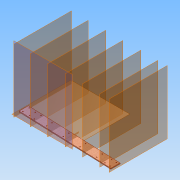
# Autodesk Inventor part: Pancake_Timing Backboard 2
Saved by Autodesk Inventor 2018.1 (Build 221171000, 171)
## iProperties
Created: 2019-02-22
Part Number: Pancake_Timing Backboard 2
Material: Wood (Oak)
Document SubType Name: Modeling
Designer: James
Density: 0.76 g/cm^3
Appearance: White Oak - Natural Medium Gloss
Author: James
Autodesk Inventor part; units mm, degrees
ref_plane "YZ Plane" through (0, 0, 0) normal (1, 0, 0) x (0, 1, 0)
ref_plane "XZ Plane" through (0, 0, 0) normal (0, 1, 0) x (-1, 0, 0)
ref_plane "XY Plane" through (0, 0, 0) normal (0, 0, 1) x (1, 0, 0)
derived "Pancake_Skeleton.ipt"
ref_plane "Ground" through (0, 0, 0) normal (0, 1, 0) x (-1, 0, 0)
ref_plane "Back" through (0, 0, 0) normal (0, 0, 1) x (1, 0, 0)
ref_plane "LHS" through (0, 0, 0) normal (1, 0, 0) x (0, 1, 0)
ref_plane "Lane 1" through (90, 0, 0) normal (1, 0, 0) x (0, 1, 0)
ref_plane "Lane 2" through (185, 0, 0) normal (1, 0, 0) x (0, 1, 0)
ref_plane "Lane 3" through (280, 0, 0) normal (1, 0, 0) x (0, 1, 0)
ref_plane "Lane 4" through (375, 0, 0) normal (1, 0, 0) x (0, 1, 0)
ref_plane "Lane 5" through (470, 0, 0) normal (1, 0, 0) x (0, 1, 0)
ref_plane "RHS" through (520, 0, 0) normal (1, 0, 0) x (0, 1, 0)
sketch "Sketch1" plane through (0, 0, 0) normal (0, 0, 1) x (1, 0, 0)
  line L0 (0, 84) -> (0, -14) projected
  line L1 (520, 84) -> (520, -14) projected
  line L2 (0, 20) -> (520, 0)
  line L3 (520, 0) -> (520, 50)
  line L4 (520, 50) -> (0, 70)
  line L5 (0, 70) -> (0, 20)
  line L6 (-104, 0) -> (624, 0) projected
  dimension "d31" = 50
  dimension "d32" = 20
  constraints: 8 end point, 2 parallel, 2 point on line, 1 collinear, 1 vertical
  measures "d31" distance of L2.end L3.end
  measures "d32" vertical distance of L2.end L2.start
extrude "Extrusion1" add sketch "Sketch1" along normal blind 5 contours L4 L1 L2 L0
sketch "Sketch2" plane through (0, 0, 5) normal (0, 0, 1) x (1, 0, 0)
  line L0 (90, 84) -> (90, -14) projected
  line L1 (520, 50) -> (0, 70) projected
  line L2 (-104, 0) -> (624, 0) projected
  line L3 (185, 96) -> (185, -16) projected
  line L4 (0, 96) -> (0, -16) projected
  line L5 (0, 20) -> (520, 0) projected
  point P0 (0, 0)
  point P1 (50, 58.0769)
  point P2 (50, 28.0769)
  dimension "d4" = 30
  dimension "d29" = 95
  dimension "d30" = 50
  dimension "d33" = 9.9926
  dimension "d34" = 9.9926
  constraints: 1 vertical alignment
  measures "d4" distance of point (50, 28.077) point (50, 58.077)
  measures "d29" distance between parallel lines of L3 L0
  measures "d30" distance from line of point (50, 58.077) L4
  measures "d33" distance from line of L1 point (50, 58.077)
  measures "d34" distance from line of L5 point (50, 28.077)
hole "Hole1" at (50, 58.0769, 5) at (50, 28.0769, 5) direction (0, 0, -1) diameter 4.5 end through all clearance for "Socket Head Cap Screw" size "M4" standard "Ansi Metric M Profile"
pattern_linear "Rectangular Pattern1" count 5 spacing 95 along (0.9992612, -0.0384331, 0) of "Hole1"
sketch "Sketch3" plane through (0, 0, 5) normal (0, 0, 1) x (1, 0, 0)
  line L0 (520, 50) -> (0, 70) projected
  line L1 (-104, 0) -> (624, 0) projected
  line L2 (0, 96) -> (0, -16) projected
  line L3 (0, 20) -> (520, 0) projected
  line L4 (520, 84) -> (520, -14) projected
  point P0 (0, 0)
  point P1 (12.5, 62.5)
  point P2 (12.5, 27.5)
  point P3 (507.5, 42.5)
  point P4 (507.5, 7.5)
  dimension "d20" = 12.5
  dimension "d36" = 35
  dimension "d38" = 12.5
  dimension "d39" = 35
  dimension "d41" = 7.5
  dimension "d42" = 7.5
  constraints: 2 vertical alignment
  measures "d20" distance from line of L2 point (12.5, 62.5)
  measures "d36" distance of point (12.5, 27.5) point (12.5, 62.5)
  measures "d38" distance from line of L4 point (507.5, 42.5)
  measures "d39" distance of point (507.5, 7.5) point (507.5, 42.5)
  measures "d41" vertical distance of L0.start point (507.5, 42.5)
  measures "d42" vertical distance of point (12.5, 62.5) L0.end
hole "Hole2" at (12.5, 62.5, 5) at (12.5, 27.5, 5) at (507.5, 42.5, 5) at (507.5, 7.5, 5) direction (0, 0, -1) diameter 4.5 end through all clearance for "Socket Head Cap Screw" size "M4" standard "Ansi Metric M Profile"
ref_plane "Work Plane10" through (260, 20, 0) normal (-1, 0, 0) x (0, 0, 1)
sketch "Sketch4" plane through (0, 0, 5) normal (0, 0, 1) x (1, 0, 0)
  line L0 (80, 59.4175) -> (78.6548, 24.4434)
  line L1 (479.7045, 44.0443) -> (478.3593, 9.0701)
  line L2 (520, 50) -> (0, 70) projected
  line L3 (0, 20) -> (520, 0) projected
  line L4 (0, 84) -> (0, -14) projected
  line L5 (520, 84) -> (520, -14) projected
  point P0 (0, 0)
  dimension "d43" = 7.5
  dimension "d44" = 7.5
  dimension "d48" = 35
  dimension "d49" = 80
  dimension "d58" = 35
  dimension "d60" = 400
  constraints: 4 end point, 2 perpendicular
  measures "d43" distance from line of L2 L0.start
  measures "d44" distance from line of L2 L1.start
  measures "d48" distance of L0.start L0.end
  measures "d49" distance from line of L0.start L4
  measures "d58" distance of L1.start L1.end
  measures "d60" distance of L1.start L0.start
hole "Hole3" at (80, 59.4175, 5) at (78.6548, 24.4434, 5) at (479.7045, 44.0443, 5) at (478.3593, 9.0701, 5) direction (0, 0, -1) diameter 4.5 end through all clearance for "Flat Head Machine Screw" size "M4" standard "Ansi Metric M Profile"
equation "\"d33\" = d34"
equation "\"d44\" = d43"
equation "\"d58\" = d48"
body "Solid1"
